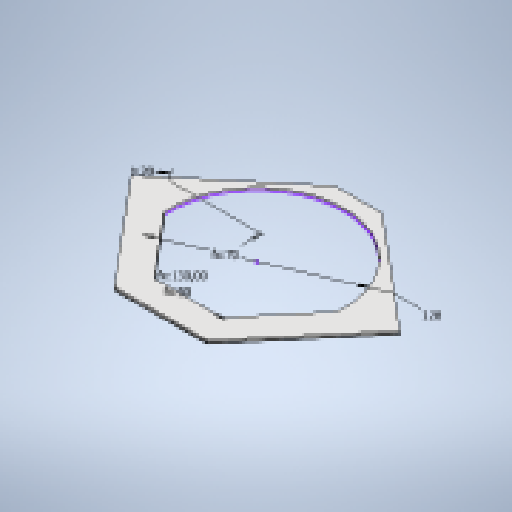
# Autodesk Inventor part: ДМФ 054 фланец лотка v2.0
Saved by Autodesk Inventor 2026.2 (Build 302298010, 298A)
## iProperties
Created: 2024-05-14
Part Number: ДМФ 054 фланец лотка v2.0
Material: Generic
Document SubType Name: Sheet Metal
Designer: admin
Density: 1 g/cm^3
Sheet Metal Rule: Default_mm
Appearance: Default
Mass: 10.0564 g
Surface Area: 111.42 cm^2
Volume: 10.0564 cm^3
Flat Pattern Width: 18.961 cm
Flat Pattern Length: 18.6303 cm
Flat Pattern Area: 353.25 cm^2
Sheet Metal Width: 189,610 mm
Sheet Metal Length: 186,303 mm
Sheet Metal Area: 35324,957 mm^2
Author: admin
Autodesk Inventor part; units mm, degrees
ref_plane "YZ Plane" through (0, 0, 0) normal (1, 0, 0) x (0, 1, 0)
ref_plane "XZ Plane" through (0, 0, 0) normal (0, 1, 0) x (-1, 0, 0)
ref_plane "XY Plane" through (0, 0, 0) normal (0, 0, 1) x (1, 0, 0)
sketch "Sketch1" plane through (0, 0, 0) normal (0, 0, 1) x (1, 0, 0)
  line L0 (-25, 0) -> (25, 0)
  line L1 (25, 0) -> (83.737, 70)
  line L2 (83.737, 70) -> (99.0579, 57.1442) construction
  line L3 (99.0579, 57.1442) -> (34.3262, -20)
  line L4 (34.3262, -20) -> (-34.3262, -20)
  line L5 (-34.3262, -20) -> (-99.0579, 57.1442)
  line L6 (-99.0579, 57.1442) -> (-83.737, 70) construction
  line L7 (-83.737, 70) -> (-25, 0)
  line L8 (0, 0) -> (0, -20) construction
  line L9 (83.737, 70) -> (24.1493, 120) construction
  line L10 (24.1493, 120) -> (-24.1493, 120)
  line L11 (-24.1493, 120) -> (-83.737, 70) construction
  circle A0 centre (0, 50) radius 64
  line L12 (99.0579, 57.1442) -> (112.5, 100)
  line L13 (112.5, 100) -> (24.1493, 120)
  line L14 (-99.0579, 57.1442) -> (-112.5, 100)
  line L15 (-112.5, 100) -> (-24.1493, 120)
  point P0 (-63.8961, 46.3546)
  point P1 (63.8961, 46.3546)
  dimension "d0" = 50
  dimension "d1" = 70
  dimension "d2" = 130
  dimension "d3" = 20
  dimension "d5" = 128
  dimension "d6" = 140
  dimension "d7" = 100
  dimension "d8" = 225
  dimension "d9" = 70
  measures "d0" distance of L0.start L0.end
  measures "d1" distance from line of L0 L6.end
  measures "d2" angle of L0 L7
  measures "d3" distance of L5.end L6.end
  measures "d5" diameter of A0
  measures "d6" distance between parallel lines of L4 L10
  measures "d7" vertical distance of L12.end point (0, 0)
  measures "d8" distance of L12.end L14.end
  measures "d9" distance from line of L4 A0.centre
extrude "Plate1" add sketch "Sketch1" along normal blind 2 contours L0 L1 A0 L7 | L3 L4 L5 L14 L15 L10 L13 L12 picked at (0, -4.6667)
equation "\"d0\" = Лоток_ширина_низ"
equation "\"d1\" = Лоток_высота - Лоток_глубина_выреза"
equation "\"d2\" = Лоток_угол"
equation "\"d4\" = Thickness"
equation "\"BendRadius\" = Thickness"
equation "\"BendReliefWidth\" = Thickness"
equation "\"BendReliefDepth\" = 0.5 * Thickness"
equation "\"CornerReliefSize\" = 4 * Thickness"
equation "\"MinimumRemnant\" = 2 * Thickness"
equation "\"TransitionRadius\" = BendRadius"
equation "\"JacobiRadiusSize\" = BendRadius"
equation "\"GapSize\" = Thickness"
equation "\"Лоток_ширина_низ\" = 50"
equation "\"Лоток_высота\" = 100"
equation "\"Лоток_глубина_выреза\" = 30"
equation "\"Лоток_угол\" = 130deg"
equation "\"Thickness\" = 2"
body "Solid1"
